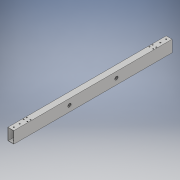
# Autodesk Inventor part: 1x1 27in
Saved by Autodesk Inventor 2018 (Build 220112000, 112)
## iProperties
Created: 2019-01-13
Part Number: 1x1 27in
Material: Generic
Document SubType Name: Modeling
Designer: s-2512711
Density: 1 g/cm^3
Appearance: Default
Mass: 157.355 g
Surface Area: 1994.16 cm^2
Volume: 157.355 cm^3
Author: s-2512711
Autodesk Inventor part; units mm, degrees
ref_plane "YZ Plane" through (0, 0, 0) normal (1, 0, 0) x (0, 1, 0)
ref_plane "XZ Plane" through (0, 0, 0) normal (0, 1, 0) x (-1, 0, 0)
ref_plane "XY Plane" through (0, 0, 0) normal (0, 0, 1) x (1, 0, 0)
sketch "Sketch1" plane through (0, 0, 0) normal (0, 0, 1) x (1, 0, 0)
  line L0 (0, 0) -> (25.4, 0)
  line L1 (25.4, 0) -> (25.4, 50.8)
  line L2 (25.4, 50.8) -> (0, 50.8)
  line L3 (0, 50.8) -> (0, 0)
  line L4 (1.5875, 1.5875) -> (23.8125, 1.5875)
  line L5 (23.8125, 1.5875) -> (23.8125, 49.2125)
  line L6 (23.8125, 49.2125) -> (1.5875, 49.2125)
  line L7 (1.5875, 49.2125) -> (1.5875, 1.5875)
  dimension "d0" = 25.4
  dimension "d1" = 50.8
  dimension "d2" = 1.5875
  constraints: 16 end point, 4 parallel, 2 perpendicular, 1 horizontal, 3 other
  measures "d0" distance of L2.end L1.end
  measures "d1" distance of L1.end L0.end
  measures "d2" distance between parallel lines of L3 L7
extrude "Extrusion1" add sketch "Sketch1" along normal blind 685.8
sketch "Sketch2" plane through (0, 50.8, 0) normal (0, 1, 0) x (1, 0, 0)
  line L0 (25.4, 0) -> (0, 0) construction
  line L1 (12.7, 0) -> (12.7, -12.7) construction
  line L2 (12.7, -12.7) -> (12.7, -38.1) construction
  line L3 (0, 0) -> (0, -685.8) construction
  line L4 (0, -342.9) -> (25.4, -342.9) construction
  circle A0 centre (12.7, -38.1) radius 2.5797
  circle A1 centre (12.7, -12.7) radius 2.5797
  line L5 (25.4, -685.8) -> (0, -685.8) construction
  line L6 (12.7, -685.8) -> (12.7, -673.1) construction
  line L7 (12.7, -673.1) -> (12.7, -647.7) construction
  line L8 (0, -685.8) -> (0, 0) construction
  circle A2 centre (12.7, -647.7) radius 2.5797
  circle A3 centre (12.7, -673.1) radius 2.5797
  dimension "d5" = 12.7
  dimension "d6" = 25.4
  dimension "d7" = 5.1594
  constraints: 14 end point, 8 symmetric about line, 4 centre point, 4 coincident, 2 midpoint, 2 point on line, 1 horizontal, 1 vertical, 2 other
  measures "d5" distance of L1.start L1.end
  measures "d6" distance of L1.end L2.end
  measures "d7" diameter of A0
extrude "Extrusion2" cut sketch "Sketch2" against normal blind 165.1
sketch "Sketch6" plane through (25.4, 0, 0) normal (1, 0, 0) x (0, 0, -1)
  line L0 (0, 50.8) -> (0, 0) construction
  line L1 (0, 25.4) -> (-241.3, 25.4) construction
  line L2 (0, 49.2125) -> (-685.8, 49.2125) construction
  line L3 (-342.9, 49.2125) -> (-342.9, -29.9468) construction
  circle A0 centre (-241.3, 25.4) radius 7.493
  circle A1 centre (-444.5, 25.4) radius 7.493
  dimension "d32" = 241.3
  dimension "d33" = 14.986
  constraints: 4 end point, 2 centre point, 2 midpoint, 1 coincident, 1 horizontal, 1 symmetric about line, 1 vertical, 1 other
  measures "d32" distance of L1.start L1.end
  measures "d33" diameter of A0
extrude "Extrusion9" cut sketch "Sketch6" against normal blind 25.4
sketch "Sketch7" plane through (0, 50.8, 0) normal (0, 1, 0) x (1, 0, 0)
  line L0 (0, 0) -> (0, -83.35) construction
  line L1 (0, 0) -> (0, -685.8) construction
  line L2 (0, -83.35) -> (0, -77) construction
  line L3 (0, -77) -> (4.75, -77) construction
  line L4 (4.75, -77) -> (20.75, -77) construction
  line L5 (20.75, -77) -> (20.75, -63.5) construction
  line L6 (20.75, -63.5) -> (4.75, -63.5) construction
  circle A0 centre (4.75, -77) radius 2.3
  circle A1 centre (4.75, -63.5) radius 2.3
  circle A2 centre (20.75, -63.5) radius 2.3
  circle A3 centre (20.75, -77) radius 2.3
  line L7 (25.4, 0) -> (25.4, -685.8) construction
  line L8 (25.4, -342.9) -> (0, -342.9) construction
  circle A4 centre (4.75, -608.8) radius 2.3
  circle A5 centre (4.75, -622.3) radius 2.3
  circle A6 centre (20.75, -622.3) radius 2.3
  circle A7 centre (20.75, -608.8) radius 2.3
  dimension "d37" = 83.35
  dimension "d38" = 6.35
  dimension "d39" = 4.75
  dimension "d40" = 16
  dimension "d41" = 13.5
  dimension "d42" = 4.6
  dimension "d45" = 4.6
  dimension "d46" = 4.6
  dimension "d47" = 4.6
  constraints: 14 end point, 8 centre point, 4 coincident, 4 symmetric about line, 3 perpendicular, 2 midpoint, 2 point on line, 1 horizontal, 4 other
  measures "d37" distance of L0.start L0.end
  measures "d38" distance of L0.end L2.end
  measures "d39" distance of L2.end L3.end
  measures "d40" distance of L3.end L4.end
  measures "d41" distance of L4.end L5.end
  measures "d42" diameter of A0
  measures "d45" diameter of A1
  measures "d46" diameter of A2
  measures "d47" diameter of A3
extrude "Extrusion10" cut sketch "Sketch7" against normal blind 100.0125
body "Solid1"
